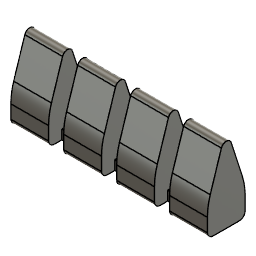
slide_potentiometer_knob (Autodesk Fusion 360 design; units mm, degrees)
Autodesk Fusion 360 part; units mm, degrees
sketch "Sketch1" plane through (0, 0, 0) normal (0, 1, 0) x (1, 0, 0)
  line L0 (0, 0) -> (10, 0)
  line L1 (10, 0) -> (10, 10)
  line L2 (10, 10) -> (0, 10)
  line L3 (0, 10) -> (0, 0)
  dimension "d1" = 10
  dimension "d2" = 10
  constraint horizontal L0
  constraint vertical L1
  constraint horizontal L2
  constraint vertical L3
  constraint coincident L0.start L3.end
  measures "d1" distance of L0.start L0.end
  measures "d2" distance of L0.start L2.end
extrude "Extrude1" add sketch "Sketch1" along normal blind 20 makes body 1
chamfer "Chamfer1" distance 4 distance2 12.5 2 edges at (5, 20, 0) (5, 20, -10) measured on face at (3.3333, 20, -6.6667) measured on face at (3.3333, 20, -6.6667) on bodies 1
fillet "Fillet1" radius 1.37 2 edges at (5, 20, -6) (5, 20, -4) on bodies 1
fillet "Fillet2" radius 15.75 2 edges at (5, 7.5, 0) (5, 7.5, -10) on bodies 1
sketch "Sketch2" plane through (0, 0, 0) normal (0, -1, 0) x (1, 0, 0)
  line L0 (0, 0) -> (0, -10)
  line L1 (0, -10) -> (10, -10)
  line L2 (10, -10) -> (10, 0)
  line L3 (10, 0) -> (0, 0)
  line L4 (4.35, -2.95) -> (5.65, -2.95)
  line L5 (5.65, -2.95) -> (5.65, -7.05)
  line L6 (5.65, -7.05) -> (4.35, -7.05)
  line L7 (4.35, -7.05) -> (4.35, -2.95)
  dimension "d11" = 1.3
  dimension "d12" = 4.1
  dimension "d13" = 4.35
  dimension "d14" = 4.35
  dimension "d15" = 2.95
  dimension "d16" = 2.95
  constraint horizontal L4
  constraint vertical L5
  constraint horizontal L6
  constraint vertical L7
  measures "d11" distance of L4.start L4.end
  measures "d12" distance of L4.start L6.end
  measures "d13" distance of L2 L5
  measures "d14" distance of L0 L7
  measures "d15" distance of L3 L4
  measures "d16" distance of L1 L6
extrude "Extrude2" cut sketch "Sketch2" against normal blind 12 contours L4 L5 L6 L7 bodies 1
chamfer "Chamfer2" distance 1 angle 45 4 edges at (5.65, 0, -5) (5, 0, -2.95) (4.35, 0, -5) (5, 0, -7.05) on bodies 1
fillet "Fillet3" radius 1.5 2 edges at (5, 0, -10) (5, 0, 0) on bodies 1
copy_body "CopyPasteBodies3" bodies 1 makes body 2
move_body "Move3" bodies 2 to x (1, 0, 0) y (0, 1, 0) z (0, 0, 1) at (-11, 0, 0)
copy_body "CopyPasteBodies4" bodies 1 2 makes body 3 makes body 4
move_body "Move4" bodies 3 4 to x (1, 0, 0) y (0, 1, 0) z (0, 0, 1) at (22, 0, 0)
move_body "Move5" bodies 3 to x (1, 0, 0) y (0, 1, 0) z (0, 0, 1) at (3, 0, 0)
move_body "Move6" bodies 1 to x (1, 0, 0) y (0, 1, 0) z (0, 0, 1) at (-3, 0, 0)
move_body "Move7" bodies 2 to x (1, 0, 0) y (0, 1, 0) z (0, 0, 1) at (-6, 0, 0)
sketch "Sketch4" plane through (25, 0, 0) normal (-1, 0, 0) x (0, 0, 1)
  arc A0 (-1.5, 0) -> (0, 1.5) centre (-1.5, 1.5) ccw
  line L0 (0, 1.5) -> (0, 5.0414)
  arc A1 (0, 5.0414) -> (-0.7493, 9.8416) centre (-15.75, 5.0414) ccw
  line L1 (-0.7493, 9.8416) -> (-3.6952, 19.0474)
  arc A2 (-3.6952, 19.0474) -> (-6.3048, 19.0475) centre (-5, 18.6299) ccw
  line L2 (-6.3048, 19.0475) -> (-6.3048, 19.0474)
  line L3 (-6.3048, 19.0474) -> (-9.2507, 9.8416)
  arc A3 (-9.2507, 9.8416) -> (-10, 5.0414) centre (5.75, 5.0414) ccw
  line L4 (-10, 5.0414) -> (-10, 1.5)
  arc A4 (-10, 1.5) -> (-8.5, 0) centre (-8.5, 1.5) ccw
  line L5 (-8.5, 0) -> (-1.5, 0)
  line L6 (-6, 0) -> (-3.5, 0)
  line L7 (-3.5, 0) -> (-3.5, 2.5)
  line L8 (-3.5, 2.5) -> (-6, 2.5)
  line L9 (-6, 2.5) -> (-6, 0)
  dimension "d22" = 2.5
  constraint perpendicular L6 L7
  constraint parallel L6 L8
  constraint parallel L7 L9
  constraint coincident L5 L6.end
  constraint coincident L5 L6.start
  measures "d22" distance of L6.start L8.end
sketch "Sketch5" plane through (11, 0, 0) normal (-1, 0, 0) x (0, 0, 1)
  arc A0 (-1.5, 0) -> (0, 1.5) centre (-1.5, 1.5) ccw
  line L0 (0, 1.5) -> (0, 5.0414)
  arc A1 (0, 5.0414) -> (-0.7493, 9.8416) centre (-15.75, 5.0414) ccw
  line L1 (-0.7493, 9.8416) -> (-3.6952, 19.0474)
  arc A2 (-3.6952, 19.0474) -> (-6.3048, 19.0475) centre (-5, 18.6299) ccw
  line L2 (-6.3048, 19.0475) -> (-6.3048, 19.0474)
  line L3 (-6.3048, 19.0474) -> (-9.2507, 9.8416)
  arc A3 (-9.2507, 9.8416) -> (-10, 5.0414) centre (5.75, 5.0414) ccw
  line L4 (-10, 5.0414) -> (-10, 1.5)
  arc A4 (-10, 1.5) -> (-8.5, 0) centre (-8.5, 1.5) ccw
  line L5 (-8.5, 0) -> (-1.5, 0)
  line L6 (-6, 0) -> (-3.5, 0)
  line L7 (-3.5, 0) -> (-3.5, 2.5)
  line L8 (-3.5, 2.5) -> (-6, 2.5)
  line L9 (-6, 2.5) -> (-6, 0)
  constraint horizontal L6
  constraint vertical L7
  constraint horizontal L8
  constraint vertical L9
  constraint coincident L5 L6.start
sketch "Sketch6" plane through (-3, 0, 0) normal (-1, 0, 0) x (0, 0, 1)
  arc A0 (-1.5, 0) -> (0, 1.5) centre (-1.5, 1.5) ccw
  line L0 (0, 1.5) -> (0, 5.0414)
  arc A1 (0, 5.0414) -> (-0.7493, 9.8416) centre (-15.75, 5.0414) ccw
  line L1 (-0.7493, 9.8416) -> (-3.6952, 19.0474)
  arc A2 (-3.6952, 19.0474) -> (-6.3048, 19.0475) centre (-5, 18.6299) ccw
  line L2 (-6.3048, 19.0475) -> (-6.3048, 19.0474)
  line L3 (-6.3048, 19.0474) -> (-9.2507, 9.8416)
  arc A3 (-9.2507, 9.8416) -> (-10, 5.0414) centre (5.75, 5.0414) ccw
  line L4 (-10, 5.0414) -> (-10, 1.5)
  arc A4 (-10, 1.5) -> (-8.5, 0) centre (-8.5, 1.5) ccw
  line L5 (-8.5, 0) -> (-1.5, 0)
  line L6 (-6, 0) -> (-3.5, 0)
  line L7 (-3.5, 0) -> (-3.5, 2.5)
  line L8 (-3.5, 2.5) -> (-6, 2.5)
  line L9 (-6, 2.5) -> (-6, 0)
  constraint horizontal L6
  constraint vertical L7
  constraint horizontal L8
  constraint vertical L9
  constraint coincident L5 L6.start
extrude "Extrude3" add sketch "Sketch4" along normal blind 4 contours L5 L6 L7 L8 L9 bodies 3 4
extrude "Extrude4" add sketch "Sketch5" along normal blind 4 contours L5 L6 L7 L8 L9 bodies 1 3
extrude "Extrude5" add sketch "Sketch6" along normal blind 4 contours L5 L6 L7 L8 L9 bodies 1 2
